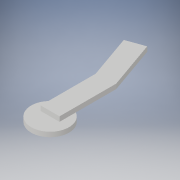
# Autodesk Inventor part: scale_l_arm
Saved by Autodesk Inventor 2018 (Build 220112000, 112)
## iProperties
Created: 2018-05-04
Part Number: scale_l_arm
Material: Generic
Document SubType Name: Modeling
Designer: 4070609
Density: 1 g/cm^3
Appearance: Default
Author: 4070609
Autodesk Inventor part; units mm, degrees
ref_plane "YZ Plane" through (0, 0, 0) normal (1, 0, 0) x (0, 1, 0)
ref_plane "XZ Plane" through (0, 0, 0) normal (0, 1, 0) x (-1, 0, 0)
ref_plane "XY Plane" through (0, 0, 0) normal (0, 0, 1) x (1, 0, 0)
sketch "Sketch1" plane through (0, 0, 0) normal (0, 1, 0) x (-1, 0, 0)
  circle A0 centre (0, 0) radius 20
  dimension "d0" = 40
  constraints: 1 centre point, 1 coincident
  measures "d0" diameter of A0
extrude "Extrusion1" add sketch "Sketch1" along normal blind 5
sketch "Sketch2" plane through (0, 5, 0) normal (0, 1, 0) x (1, 0, 0)
  line L0 (0, 0) -> (0, 60)
  line L1 (0, 60) -> (-17.2323, 107.3454)
  line L2 (10, 0) -> (-10, 0)
  line L3 (-10, 0) -> (-10, 60)
  line L4 (-10, 60) -> (10, 60)
  line L5 (10, 60) -> (10, 0)
  line L6 (10, 0) -> (-10, 60) construction
  line L7 (-10, 0) -> (10, 60) construction
  line L8 (-17.2323, 107.3454) -> (-7.8354, 110.7656)
  line L9 (-7.8354, 110.7656) -> (10, 60)
  line L10 (0, 60) -> (-9.3969, 56.5798)
  line L11 (-9.3969, 56.5798) -> (-26.0986, 104.1184)
  line L12 (-26.0986, 104.1184) -> (-17.2323, 107.3454)
  point P0 (0, 30)
  dimension "d3" = 60
  dimension "d4" = 160
  dimension "d5" = 20
  dimension "d6" = 60
  dimension "d9" = 10
  dimension "d10" = 10
  constraints: 26 end point, 3 midpoint, 2 parallel, 2 perpendicular, 1 horizontal, 1 vertical
  measures "d3" distance of L0.start L0.end
  measures "d4" angle of L1 L0
  measures "d5" distance of L3.end L4.end
  measures "d6" distance of L2.end L3.end
  measures "d9" distance of L1.end L8.end
  measures "d10" distance of L0.end L10.end
extrude "Extrusion2" add sketch "Sketch2" along normal blind 5 contours L2 L3 L11 L10 L0 | L0 L4 L5 L2 | L4 L3 L11 L12 L1 | L10 L11 L3 L4
sketch "Sketch3" plane through (0, 10, 0) normal (0, 1, 0) x (1, 0, 0)
  line L0 (0, 60) -> (-17.2323, 107.3454) projected
  line L1 (-17.2323, 107.3454) -> (-26.0986, 104.1184) projected
  line L2 (-17.2323, 107.3454) -> (-7.7976, 110.66)
  line L3 (10, 60) -> (0, 60) projected
  line L4 (-7.7976, 110.66) -> (10, 60)
  line L5 (0, 60) -> (-17.2323, 107.3454) projected
  line L6 (10, 60) -> (0, 60)
  line L7 (0, 60) -> (-17.2323, 107.3454)
  point P0 (0, 0)
  dimension "d13" = 10
  constraints: 8 end point, 1 collinear, 1 horizontal, 1 perpendicular
  measures "d13" distance of L0.end L2.end
extrude "Extrusion3" add sketch "Sketch3" against normal blind 5
body "Solid1"
